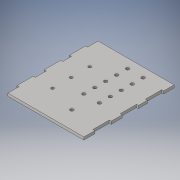
# Autodesk Inventor part: Frontpanel
Saved by Autodesk Inventor 2016 (Build 200138000, 138)
## iProperties
Created: 2016-05-17
Part Number: Frontpanel
Material: Generic
Document SubType Name: Modeling
Designer: Lillahunden
Density: 1 g/cm^3
Appearance: Default
Mass: 190.183 g
Surface Area: 679.872 cm^2
Volume: 190.183 cm^3
Author: Lillahunden
Autodesk Inventor part; units mm, degrees
ref_plane "YZ Plane" through (0, 0, 0) normal (1, 0, 0) x (0, 1, 0)
ref_plane "XZ Plane" through (0, 0, 0) normal (0, 1, 0) x (-1, 0, 0)
ref_plane "XY Plane" through (0, 0, 0) normal (0, 0, 1) x (1, 0, 0)
sketch "Sketch1" plane through (0, 0, 0) normal (0, 0, 1) x (1, 0, 0)
  line L0 (189.5387, -1221.4231) -> (189.5387, -1249.7948) projected
  line L1 (189.5387, -1249.7948) -> (185.3914, -1249.7948) projected
  line L2 (185.3914, -1227.4231) -> (26.2531, -1227.4231) projected
  line L3 (189.5387, -1227.4231) -> (185.3914, -1227.4231) projected
  line L4 (185.3914, -1249.7948) -> (185.3914, -1284.7948) projected
  line L5 (185.3914, -1284.7948) -> (189.5387, -1284.7948) projected
  line L6 (189.5387, -1284.7948) -> (189.5387, -1303.9231) projected
  line L7 (189.5387, -1303.9231) -> (185.3914, -1303.9231) projected
  line L8 (185.3914, -1303.9231) -> (185.3914, -1338.9231) projected
  line L9 (189.5387, -1338.9231) -> (189.5387, -1362.6731) projected
  line L10 (185.3914, -1338.9231) -> (189.5387, -1338.9231) projected
  line L11 (189.5387, -1362.6731) -> (185.3914, -1362.6731) projected
  line L12 (185.3914, -1362.6731) -> (185.3914, -1397.6731) projected
  line L13 (185.3914, -1397.6731) -> (189.5387, -1397.6731) projected
  line L14 (189.5387, -1397.6731) -> (189.5387, -1421.4231) projected
  line L15 (189.5387, -1421.4231) -> (185.3914, -1421.4231) projected
  line L16 (185.3914, -1421.4231) -> (26.2531, -1421.4231) projected
  line L17 (26.2531, -1415.4231) -> (26.2531, -1421.4231) projected
  line L18 (26.2531, -1421.4231) -> (26.2531, -1397.6731) projected
  line L19 (26.2531, -1397.6731) -> (21.9172, -1397.6731) projected
  line L20 (21.9172, -1397.6731) -> (21.9172, -1362.6731) projected
  line L21 (21.9172, -1362.6731) -> (26.2531, -1362.6731) projected
  line L22 (26.2531, -1362.6731) -> (26.2531, -1338.9231) projected
  line L23 (26.2531, -1338.9231) -> (21.9172, -1338.9231) projected
  line L24 (21.9172, -1338.9231) -> (21.9172, -1303.9231) projected
  line L25 (21.9172, -1303.9231) -> (26.2531, -1303.9231) projected
  line L26 (26.2531, -1303.9231) -> (26.2531, -1284.7948) projected
  line L27 (26.2531, -1284.7948) -> (21.9172, -1284.7948) projected
  line L28 (21.9172, -1284.7948) -> (21.9172, -1249.7948) projected
  line L29 (21.9172, -1249.7948) -> (26.2531, -1249.7948) projected
  line L30 (26.2531, -1249.7948) -> (26.2531, -1221.4231) projected
  line L31 (-159.1383, -1249.7948) -> (-159.1383, -1221.4231)
  point P0 (0, 0)
  constraints: 5 other
extrude "Extrusion1" add sketch "Sketch1" against normal blind 6
sketch "Sketch2" plane through (0, 0, 0) normal (0, 0, 1) x (1, 0, 0)
  circle A0 centre (109.5387, -1341.4231) radius 3.55
  line L0 (26.2531, -1421.4231) -> (189.5387, -1421.4231) projected
  line L1 (21.9172, -1362.6731) -> (21.9172, -1397.6731) projected
  line L2 (189.5387, -1421.4231) -> (189.5387, -1397.6731) projected
  point P0 (0, 0)
  dimension "d2" = 7.1
  dimension "d3" = 80
  dimension "d13" = 80
  constraints: 1 centre point
  measures "d2" diameter of A0
  measures "d3" distance from line of L0 A0.centre
  measures "d13" distance from line of L2 A0.centre
extrude "Extrusion2" cut sketch "Sketch2" against normal through all
pattern_linear "Rectangular Pattern1" count 5 spacing 23.5 along (0, 1, 0) count 2 spacing 33.5 along (1, 0, 0) of "Extrusion2"
sketch "Sketch3" plane through (0, 0, 0) normal (0, 0, 1) x (1, 0, 0)
  circle A0 centre (143.0387, -1341.4231) radius 3.55 construction
  circle A1 centre (109.5387, -1341.4231) radius 3.55 construction
  line L0 (143.0387, -1341.4231) -> (109.5387, -1341.4231) construction
  line L1 (126.2887, -1341.4231) -> (126.2887, -1398.6918) construction
  circle A2 centre (126.2887, -1383.9944) radius 3.6
  point P0 (0, 0)
  dimension "d14" = 7.2
  constraints: 4 end point, 1 centre point, 1 horizontal, 1 midpoint, 1 point on line, 1 vertical
  measures "d14" diameter of A2
extrude "Extrusion3" cut sketch "Sketch3" against normal through all
sketch "Sketch4" plane through (0, 0, 0) normal (0, 0, 1) x (1, 0, 0)
  circle A0 centre (65.2908, -1284.4231) radius 3.1
  line L0 (189.5387, -1227.4231) -> (26.2531, -1227.4231) projected
  circle A1 centre (65.2908, -1324.4231) radius 3.1
  circle A2 centre (65.2908, -1364.4231) radius 3.1
  line L1 (26.2531, -1421.4231) -> (189.5387, -1421.4231) projected
  point P0 (0, 0)
  dimension "d17" = 6.2
  dimension "d18" = 57
  dimension "d19" = 6.2
  dimension "d20" = 6.2
  dimension "d21" = 40
  dimension "d22" = 40
  dimension "d23" = 57
  constraints: 3 centre point, 2 vertical alignment
  measures "d17" diameter of A0
  measures "d18" distance from line of L0 A0.centre
  measures "d19" diameter of A1
  measures "d20" diameter of A2
  measures "d21" distance of A1.centre A0.centre
  measures "d22" distance of A1.centre A2.centre
  measures "d23" distance from line of L1 A2.centre
extrude "Extrusion4" cut sketch "Sketch4" against normal through all
body "Solid1"
